Autodesk Fusion 360 part; units mm, degrees
(part 3 of 18)
  line L1811 (74.8364, -20.1454) -> (75.1219, -20.8347)
  line L1812 (79.0262, -16.9304) -> (78.3369, -16.6449)
  line L1813 (74.739, -19.4056) -> (74.8364, -20.1454)
  line L1814 (76.1681, -16.9304) -> (75.5761, -17.3846)
  line L1815 (80.3579, -18.6659) -> (80.0724, -17.9766)
  line L1816 (75.1219, -20.8347) -> (75.5761, -21.4267)
  line L1817 (78.3369, -16.6449) -> (77.5972, -16.5475)
  line L1818 (79.6182, -17.3846) -> (79.0262, -16.9304)
  line L1819 (75.1219, -17.9766) -> (74.8364, -18.6659)
  line L1820 (77.5972, -22.2638) -> (78.3369, -22.1664)
  line L1821 (75.5761, -21.4267) -> (76.1681, -21.8809)
  line L1822 (76.8574, -16.6449) -> (76.1681, -16.9304)
  line L1823 (80.3579, -20.1454) -> (80.4553, -19.4056)
  line L1824 (76.8574, -22.1664) -> (77.5972, -22.2638)
  line L1825 (76.1681, -21.8809) -> (76.8574, -22.1664)
  line L1826 (76.1681, -79.0564) -> (76.8574, -79.3419)
  line L1827 (80.3579, -75.8414) -> (80.0724, -75.1521)
  line L1828 (79.6182, -78.6022) -> (80.0724, -78.0102)
  line L1829 (79.0262, -79.0564) -> (79.6182, -78.6022)
  line L1830 (78.3369, -73.8204) -> (77.5972, -73.723)
  line L1831 (79.6182, -74.5601) -> (79.0262, -74.1059)
  line L1832 (74.739, -76.5812) -> (74.8364, -77.3209)
  line L1833 (76.1681, -74.1059) -> (75.5761, -74.5601)
  line L1834 (75.1219, -78.0102) -> (75.5761, -78.6022)
  line L1835 (74.8364, -77.3209) -> (75.1219, -78.0102)
  line L1836 (80.0724, -75.1521) -> (79.6182, -74.5601)
  line L1837 (80.4553, -76.5812) -> (80.3579, -75.8414)
  line L1838 (75.5761, -78.6022) -> (76.1681, -79.0564)
  line L1839 (80.3579, -77.3209) -> (80.4553, -76.5812)
  line L1840 (80.0724, -78.0102) -> (80.3579, -77.3209)
  line L1841 (75.1219, -75.1521) -> (74.8364, -75.8414)
  line L1842 (79.0262, -74.1059) -> (78.3369, -73.8204)
  line L1843 (77.5972, -79.4393) -> (78.3369, -79.3419)
  line L1844 (76.8574, -73.8204) -> (76.1681, -74.1059)
  line L1845 (74.8364, -75.8414) -> (74.739, -76.5812)
  line L1846 (75.5761, -74.5601) -> (75.1219, -75.1521)
  line L1847 (77.5972, -73.723) -> (76.8574, -73.8204)
  line L1848 (76.8574, -79.3419) -> (77.5972, -79.4393)
  line L1849 (78.3369, -79.3419) -> (79.0262, -79.0564)
  line L1850 (80.0724, -39.8847) -> (80.3579, -39.1954)
  line L1851 (76.1681, -35.9805) -> (75.5761, -36.4347)
  line L1852 (74.8364, -37.7159) -> (74.739, -38.4557)
  line L1853 (76.8574, -35.6949) -> (76.1681, -35.9805)
  line L1854 (80.4553, -38.4557) -> (80.3579, -37.7159)
  line L1855 (75.5761, -36.4347) -> (75.1219, -37.0266)
  line L1856 (75.1219, -37.0266) -> (74.8364, -37.7159)
  line L1857 (75.1219, -39.8847) -> (75.5761, -40.4767)
  line L1858 (79.0262, -40.9309) -> (79.6182, -40.4767)
  line L1859 (80.3579, -39.1954) -> (80.4553, -38.4557)
  line L1860 (80.3579, -37.7159) -> (80.0724, -37.0266)
  line L1861 (76.8574, -41.2164) -> (77.5972, -41.3138)
  line L1862 (77.5972, -35.5975) -> (76.8574, -35.6949)
  line L1863 (79.0262, -35.9805) -> (78.3369, -35.6949)
  line L1864 (77.5972, -41.3138) -> (78.3369, -41.2164)
  line L1865 (75.5761, -40.4767) -> (76.1681, -40.9309)
  line L1866 (78.3369, -41.2164) -> (79.0262, -40.9309)
  line L1867 (79.6182, -40.4767) -> (80.0724, -39.8847)
  line L1868 (78.3369, -35.6949) -> (77.5972, -35.5975)
  line L1869 (80.0724, -37.0266) -> (79.6182, -36.4347)
  line L1870 (79.6182, -36.4347) -> (79.0262, -35.9805)
  line L1871 (74.739, -38.4557) -> (74.8364, -39.1954)
  line L1872 (74.8364, -39.1954) -> (75.1219, -39.8847)
  line L1873 (76.1681, -40.9309) -> (76.8574, -41.2164)
  line L1874 (74.8364, -58.2582) -> (75.1219, -58.9475)
  line L1875 (79.0262, -59.9936) -> (79.6182, -59.5394)
  line L1876 (74.8364, -56.7787) -> (74.739, -57.5184)
  line L1877 (80.3579, -58.2582) -> (80.4553, -57.5184)
  line L1878 (79.6182, -59.5394) -> (80.0724, -58.9475)
  line L1879 (76.1681, -55.0432) -> (75.5761, -55.4974)
  line L1880 (75.1219, -58.9475) -> (75.5761, -59.5394)
  line L1881 (80.0724, -58.9475) -> (80.3579, -58.2582)
  line L1882 (74.739, -57.5184) -> (74.8364, -58.2582)
  line L1883 (75.1219, -56.0893) -> (74.8364, -56.7787)
  line L1884 (76.8574, -54.7577) -> (76.1681, -55.0432)
  line L1885 (78.3369, -54.7577) -> (77.5972, -54.6603)
  line L1886 (79.0262, -55.0432) -> (78.3369, -54.7577)
  line L1887 (75.5761, -55.4974) -> (75.1219, -56.0893)
  line L1888 (75.5761, -59.5394) -> (76.1681, -59.9936)
  line L1889 (77.5972, -54.6603) -> (76.8574, -54.7577)
  line L1890 (78.3369, -60.2792) -> (79.0262, -59.9936)
  line L1891 (77.5972, -60.3766) -> (78.3369, -60.2792)
  line L1892 (80.4553, -57.5184) -> (80.3579, -56.7787)
  line L1893 (80.3579, -56.7787) -> (80.0724, -56.0893)
  line L1894 (80.0724, -56.0893) -> (79.6182, -55.4974)
  line L1895 (79.6182, -55.4974) -> (79.0262, -55.0432)
  line L1896 (76.1681, -59.9936) -> (76.8574, -60.2792)
  line L1897 (76.8574, -60.2792) -> (77.5972, -60.3766)
  line L1898 (76.4348, -83.0626) -> (76.7075, -83.4708)
  line L1899 (76.4348, -82.0997) -> (76.339, -82.5812)
  line L1900 (76.7075, -81.6915) -> (76.4348, -82.0997)
  line L1901 (76.7075, -83.4708) -> (77.1157, -83.7435)
  line L1902 (78.0786, -81.4188) -> (77.5972, -81.323)
  line L1903 (77.1157, -83.7435) -> (77.5972, -83.8393)
  line L1904 (78.0786, -83.7435) -> (78.4868, -83.4708)
  line L1905 (78.4868, -83.4708) -> (78.7595, -83.0626)
  line L1906 (76.339, -82.5812) -> (76.4348, -83.0626)
  line L1907 (78.4868, -81.6915) -> (78.0786, -81.4188)
  line L1908 (78.7595, -82.0997) -> (78.4868, -81.6915)
  line L1909 (78.7595, -83.0626) -> (78.8553, -82.5812)
  line L1910 (77.1157, -81.4188) -> (76.7075, -81.6915)
  line L1911 (77.5972, -81.323) -> (77.1157, -81.4188)
  line L1912 (77.5972, -83.8393) -> (78.0786, -83.7435)
  line L1913 (78.8553, -82.5812) -> (78.7595, -82.0997)
  line L1914 (77.5972, -62.2603) -> (77.1157, -62.3561)
  line L1915 (76.4348, -63.037) -> (76.339, -63.5184)
  line L1916 (77.1157, -62.3561) -> (76.7075, -62.6288)
  line L1917 (78.0786, -62.3561) -> (77.5972, -62.2603)
  line L1918 (78.0786, -64.6808) -> (78.4868, -64.4081)
  line L1919 (78.8553, -63.5184) -> (78.7595, -63.037)
  line L1920 (76.339, -63.5184) -> (76.4348, -63.9999)
  line L1921 (76.7075, -62.6288) -> (76.4348, -63.037)
  line L1922 (78.7595, -63.037) -> (78.4868, -62.6288)
  line L1923 (77.1157, -64.6808) -> (77.5972, -64.7766)
  line L1924 (78.4868, -64.4081) -> (78.7595, -63.9999)
  line L1925 (78.4868, -62.6288) -> (78.0786, -62.3561)
  line L1926 (76.7075, -64.4081) -> (77.1157, -64.6808)
  line L1927 (78.7595, -63.9999) -> (78.8553, -63.5184)
  line L1928 (77.5972, -64.7766) -> (78.0786, -64.6808)
  line L1929 (76.4348, -63.9999) -> (76.7075, -64.4081)
  line L1930 (77.5972, -24.1475) -> (77.1157, -24.2433)
  line L1931 (76.7075, -24.516) -> (76.4348, -24.9242)
  line L1932 (78.7595, -24.9242) -> (78.4868, -24.516)
  line L1933 (78.7595, -25.8871) -> (78.8553, -25.4057)
  line L1934 (78.8553, -25.4057) -> (78.7595, -24.9242)
  line L1935 (77.1157, -24.2433) -> (76.7075, -24.516)
  line L1936 (77.5972, -26.6638) -> (78.0786, -26.568)
  line L1937 (76.4348, -25.8871) -> (76.7075, -26.2953)
  line L1938 (78.4868, -24.516) -> (78.0786, -24.2433)
  line L1939 (78.4868, -26.2953) -> (78.7595, -25.8871)
  line L1940 (76.339, -25.4057) -> (76.4348, -25.8871)
  line L1941 (78.0786, -24.2433) -> (77.5972, -24.1475)
  line L1942 (77.1157, -26.568) -> (77.5972, -26.6638)
  line L1943 (76.4348, -24.9242) -> (76.339, -25.4057)
  line L1944 (78.0786, -26.568) -> (78.4868, -26.2953)
  line L1945 (76.7075, -26.2953) -> (77.1157, -26.568)
  line L1946 (78.0786, -43.2933) -> (77.5972, -43.1975)
  line L1947 (77.1157, -43.2933) -> (76.7075, -43.566)
  line L1948 (76.7075, -45.3453) -> (77.1157, -45.6181)
  line L1949 (76.4348, -43.9742) -> (76.339, -44.4557)
  line L1950 (78.8553, -44.4557) -> (78.7595, -43.9742)
  line L1951 (76.339, -44.4557) -> (76.4348, -44.9372)
  line L1952 (76.4348, -44.9372) -> (76.7075, -45.3453)
  line L1953 (78.4868, -45.3453) -> (78.7595, -44.9372)
  line L1954 (77.5972, -45.7138) -> (78.0786, -45.6181)
  line L1955 (78.0786, -45.6181) -> (78.4868, -45.3453)
  line L1956 (78.7595, -44.9372) -> (78.8553, -44.4557)
  line L1957 (78.7595, -43.9742) -> (78.4868, -43.566)
  line L1958 (76.7075, -43.566) -> (76.4348, -43.9742)
  line L1959 (78.4868, -43.566) -> (78.0786, -43.2933)
  line L1960 (77.5972, -43.1975) -> (77.1157, -43.2933)
  line L1961 (77.1157, -45.6181) -> (77.5972, -45.7138)
  line L1962 (99.408, -20.1454) -> (99.5053, -19.4056)
  line L1963 (97.3869, -16.6449) -> (96.6472, -16.5475)
  line L1964 (99.5053, -19.4056) -> (99.408, -18.6659)
  line L1965 (93.789, -19.4056) -> (93.8864, -20.1454)
  line L1966 (96.6472, -22.2638) -> (97.3869, -22.1664)
  line L1967 (94.172, -17.9766) -> (93.8864, -18.6659)
  line L1968 (93.8864, -20.1454) -> (94.172, -20.8347)
  line L1969 (95.2181, -21.8809) -> (95.9075, -22.1664)
  line L1970 (99.408, -18.6659) -> (99.1224, -17.9766)
  line L1971 (93.8864, -18.6659) -> (93.789, -19.4056)
  line L1972 (99.1224, -17.9766) -> (98.6682, -17.3846)
  line L1973 (96.6472, -16.5475) -> (95.9075, -16.6449)
  line L1974 (94.172, -20.8347) -> (94.6262, -21.4267)
  line L1975 (97.3869, -22.1664) -> (98.0763, -21.8809)
  line L1976 (98.0763, -16.9304) -> (97.3869, -16.6449)
  line L1977 (95.9075, -16.6449) -> (95.2181, -16.9304)
  line L1978 (98.6682, -17.3846) -> (98.0763, -16.9304)
  line L1979 (99.1224, -20.8347) -> (99.408, -20.1454)
  line L1980 (94.6262, -21.4267) -> (95.2181, -21.8809)
  line L1981 (94.6262, -17.3846) -> (94.172, -17.9766)
  line L1982 (95.2181, -16.9304) -> (94.6262, -17.3846)
  line L1983 (95.9075, -22.1664) -> (96.6472, -22.2638)
  line L1984 (98.6682, -21.4267) -> (99.1224, -20.8347)
  line L1985 (98.0763, -21.8809) -> (98.6682, -21.4267)
  line L1986 (95.9075, -73.8204) -> (95.2181, -74.1059)
  line L1987 (96.6472, -73.723) -> (95.9075, -73.8204)
  line L1988 (95.2181, -74.1059) -> (94.6262, -74.5601)
  line L1989 (95.2181, -79.0564) -> (95.9075, -79.3419)
  line L1990 (96.6472, -79.4393) -> (97.3869, -79.3419)
  line L1991 (99.1224, -78.0102) -> (99.408, -77.3209)
  line L1992 (97.3869, -79.3419) -> (98.0763, -79.0564)
  line L1993 (94.6262, -78.6022) -> (95.2181, -79.0564)
  line L1994 (93.789, -76.5812) -> (93.8864, -77.3209)
  line L1995 (99.408, -77.3209) -> (99.5053, -76.5812)
  line L1996 (94.6262, -74.5601) -> (94.172, -75.1521)
  line L1997 (93.8864, -77.3209) -> (94.172, -78.0102)
  line L1998 (98.0763, -79.0564) -> (98.6682, -78.6022)
  line L1999 (93.8864, -75.8414) -> (93.789, -76.5812)
  line L2000 (98.6682, -78.6022) -> (99.1224, -78.0102)
  line L2001 (95.9075, -79.3419) -> (96.6472, -79.4393)
  line L2002 (98.0763, -74.1059) -> (97.3869, -73.8204)
  line L2003 (99.1224, -75.1521) -> (98.6682, -74.5601)
  line L2004 (94.172, -75.1521) -> (93.8864, -75.8414)
  line L2005 (97.3869, -73.8204) -> (96.6472, -73.723)
  line L2006 (99.5053, -76.5812) -> (99.408, -75.8414)
  line L2007 (94.172, -78.0102) -> (94.6262, -78.6022)
  line L2008 (98.6682, -74.5601) -> (98.0763, -74.1059)
  line L2009 (99.408, -75.8414) -> (99.1224, -75.1521)
  line L2010 (93.8864, -39.1954) -> (94.172, -39.8847)
  line L2011 (97.3869, -35.6949) -> (96.6472, -35.5975)
  line L2012 (98.0763, -35.9805) -> (97.3869, -35.6949)
  line L2013 (98.6682, -36.4347) -> (98.0763, -35.9805)
  line L2014 (97.3869, -41.2164) -> (98.0763, -40.9309)
  line L2015 (99.5053, -38.4557) -> (99.408, -37.7159)
  line L2016 (93.8864, -37.7159) -> (93.789, -38.4557)
  line L2017 (93.789, -38.4557) -> (93.8864, -39.1954)
  line L2018 (94.172, -37.0266) -> (93.8864, -37.7159)
  line L2019 (95.9075, -35.6949) -> (95.2181, -35.9805)
  line L2020 (94.6262, -40.4767) -> (95.2181, -40.9309)
  line L2021 (96.6472, -35.5975) -> (95.9075, -35.6949)
  line L2022 (95.2181, -35.9805) -> (94.6262, -36.4347)
  line L2023 (94.172, -39.8847) -> (94.6262, -40.4767)
  line L2024 (99.408, -37.7159) -> (99.1224, -37.0266)
  line L2025 (96.6472, -41.3138) -> (97.3869, -41.2164)
  line L2026 (95.2181, -40.9309) -> (95.9075, -41.2164)
  line L2027 (95.9075, -41.2164) -> (96.6472, -41.3138)
  line L2028 (99.408, -39.1954) -> (99.5053, -38.4557)
  line L2029 (94.6262, -36.4347) -> (94.172, -37.0266)
  line L2030 (99.1224, -39.8847) -> (99.408, -39.1954)
  line L2031 (98.6682, -40.4767) -> (99.1224, -39.8847)
  line L2032 (99.1224, -37.0266) -> (98.6682, -36.4347)
  line L2033 (98.0763, -40.9309) -> (98.6682, -40.4767)
  line L2034 (95.2181, -59.9936) -> (95.9075, -60.2792)
  line L2035 (99.408, -56.7787) -> (99.1224, -56.0893)
  line L2036 (93.8864, -58.2582) -> (94.172, -58.9475)
  line L2037 (98.0763, -59.9936) -> (98.6682, -59.5394)
  line L2038 (95.2181, -55.0432) -> (94.6262, -55.4974)
  line L2039 (97.3869, -60.2792) -> (98.0763, -59.9936)
  line L2040 (97.3869, -54.7577) -> (96.6472, -54.6603)
  line L2041 (94.6262, -55.4974) -> (94.172, -56.0893)
  line L2042 (93.789, -57.5184) -> (93.8864, -58.2582)
  line L2043 (99.1224, -56.0893) -> (98.6682, -55.4974)
  line L2044 (95.9075, -60.2792) -> (96.6472, -60.3766)
  line L2045 (99.1224, -58.9475) -> (99.408, -58.2582)
  line L2046 (98.6682, -55.4974) -> (98.0763, -55.0432)
  line L2047 (94.6262, -59.5394) -> (95.2181, -59.9936)
  line L2048 (96.6472, -60.3766) -> (97.3869, -60.2792)
  line L2049 (94.172, -56.0893) -> (93.8864, -56.7787)
  line L2050 (98.0763, -55.0432) -> (97.3869, -54.7577)
  line L2051 (99.5053, -57.5184) -> (99.408, -56.7787)
  line L2052 (99.408, -58.2582) -> (99.5053, -57.5184)
  line L2053 (96.6472, -54.6603) -> (95.9075, -54.7577)
  line L2054 (93.8864, -56.7787) -> (93.789, -57.5184)
  line L2055 (98.6682, -59.5394) -> (99.1224, -58.9475)
  line L2056 (94.172, -58.9475) -> (94.6262, -59.5394)
  line L2057 (95.9075, -54.7577) -> (95.2181, -55.0432)
  line L2058 (95.7576, -81.6915) -> (95.4848, -82.0997)
  line L2059 (97.9053, -82.5812) -> (97.8096, -82.0997)
  line L2060 (95.7576, -83.4708) -> (96.1657, -83.7435)
  line L2061 (97.5368, -83.4708) -> (97.8096, -83.0626)
  line L2062 (96.1657, -83.7435) -> (96.6472, -83.8393)
  line L2063 (97.8096, -83.0626) -> (97.9053, -82.5812)
  line L2064 (95.4848, -83.0626) -> (95.7576, -83.4708)
  line L2065 (97.1287, -81.4188) -> (96.6472, -81.323)
  line L2066 (97.8096, -82.0997) -> (97.5368, -81.6915)
  line L2067 (96.6472, -83.8393) -> (97.1287, -83.7435)
  line L2068 (96.1657, -81.4188) -> (95.7576, -81.6915)
  line L2069 (95.4848, -82.0997) -> (95.3891, -82.5812)
  line L2070 (95.3891, -82.5812) -> (95.4848, -83.0626)
  line L2071 (96.6472, -81.323) -> (96.1657, -81.4188)
  line L2072 (97.5368, -81.6915) -> (97.1287, -81.4188)
  line L2073 (97.1287, -83.7435) -> (97.5368, -83.4708)
  line L2074 (96.6472, -64.7766) -> (97.1287, -64.6808)
  line L2075 (95.7576, -62.6288) -> (95.4848, -63.037)
  line L2076 (97.1287, -62.3561) -> (96.6472, -62.2603)
  line L2077 (97.5368, -62.6288) -> (97.1287, -62.3561)
  line L2078 (95.3891, -63.5184) -> (95.4848, -63.9999)
  line L2079 (96.6472, -62.2603) -> (96.1657, -62.3561)
  line L2080 (97.8096, -63.9999) -> (97.9053, -63.5184)
  line L2081 (95.4848, -63.037) -> (95.3891, -63.5184)
  line L2082 (95.7576, -64.4081) -> (96.1657, -64.6808)
  line L2083 (97.9053, -63.5184) -> (97.8096, -63.037)
  line L2084 (95.4848, -63.9999) -> (95.7576, -64.4081)
  line L2085 (97.1287, -64.6808) -> (97.5368, -64.4081)
  line L2086 (97.8096, -63.037) -> (97.5368, -62.6288)
  line L2087 (96.1657, -62.3561) -> (95.7576, -62.6288)
  line L2088 (96.1657, -64.6808) -> (96.6472, -64.7766)
  line L2089 (97.5368, -64.4081) -> (97.8096, -63.9999)
  line L2090 (97.8096, -24.9242) -> (97.5368, -24.516)
  line L2091 (95.4848, -24.9242) -> (95.3891, -25.4057)
  line L2092 (95.3891, -25.4057) -> (95.4848, -25.8871)
  line L2093 (95.4848, -25.8871) -> (95.7576, -26.2953)
  line L2094 (97.9053, -25.4057) -> (97.8096, -24.9242)
  line L2095 (96.6472, -24.1475) -> (96.1657, -24.2433)
  line L2096 (95.7576, -24.516) -> (95.4848, -24.9242)
  line L2097 (97.5368, -26.2953) -> (97.8096, -25.8871)
  line L2098 (97.8096, -25.8871) -> (97.9053, -25.4057)
  line L2099 (96.1657, -24.2433) -> (95.7576, -24.516)
  line L2100 (97.1287, -26.568) -> (97.5368, -26.2953)
  line L2101 (96.6472, -26.6638) -> (97.1287, -26.568)
  line L2102 (97.1287, -24.2433) -> (96.6472, -24.1475)
  line L2103 (96.1657, -26.568) -> (96.6472, -26.6638)
  line L2104 (97.5368, -24.516) -> (97.1287, -24.2433)
  line L2105 (95.7576, -26.2953) -> (96.1657, -26.568)
  line L2106 (96.1657, -43.2933) -> (95.7576, -43.566)
  line L2107 (95.4848, -44.9372) -> (95.7576, -45.3453)
  line L2108 (95.4848, -43.9742) -> (95.3891, -44.4557)
  line L2109 (95.7576, -43.566) -> (95.4848, -43.9742)
  line L2110 (96.1657, -45.6181) -> (96.6472, -45.7138)
  line L2111 (97.1287, -45.6181) -> (97.5368, -45.3453)
  line L2112 (97.8096, -43.9742) -> (97.5368, -43.566)
  line L2113 (97.5368, -45.3453) -> (97.8096, -44.9372)
  line L2114 (96.6472, -45.7138) -> (97.1287, -45.6181)
  line L2115 (97.5368, -43.566) -> (97.1287, -43.2933)
  line L2116 (97.9053, -44.4557) -> (97.8096, -43.9742)
  line L2117 (97.1287, -43.2933) -> (96.6472, -43.1975)
  line L2118 (96.6472, -43.1975) -> (96.1657, -43.2933)
  line L2119 (95.7576, -45.3453) -> (96.1657, -45.6181)
  line L2120 (95.3891, -44.4557) -> (95.4848, -44.9372)
  line L2121 (97.8096, -44.9372) -> (97.9053, -44.4557)
  line L2122 (114.2682, -21.8809) -> (114.9575, -22.1664)
  line L2123 (113.222, -20.8347) -> (113.6762, -21.4267)
  line L2124 (112.9365, -18.6659) -> (112.8391, -19.4056)
  line L2125 (116.437, -16.6449) -> (115.6972, -16.5475)
  line L2126 (115.6972, -22.2638) -> (116.437, -22.1664)
  line L2127 (114.2682, -16.9304) -> (113.6762, -17.3846)
  line L2128 (117.1263, -21.8809) -> (117.7182, -21.4267)
  line L2129 (117.7182, -21.4267) -> (118.1725, -20.8347)
  line L2130 (117.1263, -16.9304) -> (116.437, -16.6449)
  line L2131 (115.6972, -16.5475) -> (114.9575, -16.6449)
  line L2132 (112.8391, -19.4056) -> (112.9365, -20.1454)
  line L2133 (113.222, -17.9766) -> (112.9365, -18.6659)
  line L2134 (118.1725, -17.9766) -> (117.7182, -17.3846)
  line L2135 (116.437, -22.1664) -> (117.1263, -21.8809)
  line L2136 (118.5554, -19.4056) -> (118.458, -18.6659)
  line L2137 (112.9365, -20.1454) -> (113.222, -20.8347)
  line L2138 (118.1725, -20.8347) -> (118.458, -20.1454)
  line L2139 (114.9575, -22.1664) -> (115.6972, -22.2638)
  line L2140 (113.6762, -17.3846) -> (113.222, -17.9766)
  line L2141 (113.6762, -21.4267) -> (114.2682, -21.8809)
  line L2142 (118.458, -20.1454) -> (118.5554, -19.4056)
  line L2143 (117.7182, -17.3846) -> (117.1263, -16.9304)
  line L2144 (118.458, -18.6659) -> (118.1725, -17.9766)
  line L2145 (114.9575, -16.6449) -> (114.2682, -16.9304)
  line L2146 (117.1263, -79.0564) -> (117.7182, -78.6022)
  line L2147 (113.6762, -74.5601) -> (113.222, -75.1521)
  line L2148 (118.5554, -76.5812) -> (118.458, -75.8414)
  line L2149 (117.1263, -74.1059) -> (116.437, -73.8204)
  line L2150 (114.9575, -73.8204) -> (114.2682, -74.1059)
  line L2151 (114.2682, -74.1059) -> (113.6762, -74.5601)
  line L2152 (117.7182, -78.6022) -> (118.1725, -78.0102)
  line L2153 (115.6972, -79.4393) -> (116.437, -79.3419)
  line L2154 (117.7182, -74.5601) -> (117.1263, -74.1059)
  line L2155 (118.1725, -78.0102) -> (118.458, -77.3209)
  line L2156 (112.9365, -75.8414) -> (112.8391, -76.5812)
  line L2157 (118.458, -77.3209) -> (118.5554, -76.5812)
  line L2158 (116.437, -73.8204) -> (115.6972, -73.723)
  line L2159 (113.222, -75.1521) -> (112.9365, -75.8414)
  line L2160 (118.458, -75.8414) -> (118.1725, -75.1521)
  line L2161 (113.222, -78.0102) -> (113.6762, -78.6022)
  line L2162 (113.6762, -78.6022) -> (114.2682, -79.0564)
  line L2163 (116.437, -79.3419) -> (117.1263, -79.0564)
  line L2164 (114.2682, -79.0564) -> (114.9575, -79.3419)
  line L2165 (118.1725, -75.1521) -> (117.7182, -74.5601)
  line L2166 (112.8391, -76.5812) -> (112.9365, -77.3209)
  line L2167 (115.6972, -73.723) -> (114.9575, -73.8204)
  line L2168 (114.9575, -79.3419) -> (115.6972, -79.4393)
  line L2169 (112.9365, -77.3209) -> (113.222, -78.0102)
  line L2170 (113.222, -37.0266) -> (112.9365, -37.7159)
  line L2171 (115.6972, -41.3138) -> (116.437, -41.2164)
  line L2172 (117.1263, -35.9805) -> (116.437, -35.6949)
  line L2173 (112.9365, -37.7159) -> (112.8391, -38.4557)
  line L2174 (114.9575, -41.2164) -> (115.6972, -41.3138)
  line L2175 (113.6762, -40.4767) -> (114.2682, -40.9309)
  line L2176 (117.7182, -36.4347) -> (117.1263, -35.9805)
  line L2177 (118.458, -39.1954) -> (118.5554, -38.4557)
  line L2178 (118.458, -37.7159) -> (118.1725, -37.0266)
  line L2179 (118.1725, -39.8847) -> (118.458, -39.1954)
  line L2180 (114.2682, -35.9805) -> (113.6762, -36.4347)
  line L2181 (113.222, -39.8847) -> (113.6762, -40.4767)
  line L2182 (118.5554, -38.4557) -> (118.458, -37.7159)
  line L2183 (116.437, -41.2164) -> (117.1263, -40.9309)
  line L2184 (118.1725, -37.0266) -> (117.7182, -36.4347)
  line L2185 (117.1263, -40.9309) -> (117.7182, -40.4767)
  line L2186 (117.7182, -40.4767) -> (118.1725, -39.8847)
  line L2187 (116.437, -35.6949) -> (115.6972, -35.5975)
  line L2188 (114.9575, -35.6949) -> (114.2682, -35.9805)
  line L2189 (112.9365, -39.1954) -> (113.222, -39.8847)
  line L2190 (113.6762, -36.4347) -> (113.222, -37.0266)
  line L2191 (115.6972, -35.5975) -> (114.9575, -35.6949)
  line L2192 (112.8391, -38.4557) -> (112.9365, -39.1954)
  line L2193 (114.2682, -40.9309) -> (114.9575, -41.2164)
  line L2194 (117.7182, -59.5394) -> (118.1725, -58.9475)
  line L2195 (114.2682, -55.0432) -> (113.6762, -55.4974)
  line L2196 (117.7182, -55.4974) -> (117.1263, -55.0432)
  line L2197 (118.458, -56.7787) -> (118.1725, -56.0893)
  line L2198 (112.9365, -56.7787) -> (112.8391, -57.5184)
  line L2199 (117.1263, -55.0432) -> (116.437, -54.7577)
  line L2200 (115.6972, -54.6603) -> (114.9575, -54.7577)
  line L2201 (114.9575, -54.7577) -> (114.2682, -55.0432)
  line L2202 (113.6762, -55.4974) -> (113.222, -56.0893)
  line L2203 (117.1263, -59.9936) -> (117.7182, -59.5394)
  line L2204 (116.437, -60.2792) -> (117.1263, -59.9936)
  line L2205 (114.2682, -59.9936) -> (114.9575, -60.2792)
  line L2206 (114.9575, -60.2792) -> (115.6972, -60.3766)
  line L2207 (118.1725, -56.0893) -> (117.7182, -55.4974)
  line L2208 (113.6762, -59.5394) -> (114.2682, -59.9936)
  line L2209 (112.8391, -57.5184) -> (112.9365, -58.2582)
  line L2210 (113.222, -58.9475) -> (113.6762, -59.5394)
  line L2211 (112.9365, -58.2582) -> (113.222, -58.9475)
  line L2212 (118.5554, -57.5184) -> (118.458, -56.7787)
  line L2213 (118.458, -58.2582) -> (118.5554, -57.5184)
  line L2214 (118.1725, -58.9475) -> (118.458, -58.2582)
  line L2215 (115.6972, -60.3766) -> (116.437, -60.2792)
  line L2216 (113.222, -56.0893) -> (112.9365, -56.7787)
  line L2217 (116.437, -54.7577) -> (115.6972, -54.6603)
  line L2218 (115.6972, -81.323) -> (115.2158, -81.4188)
  line L2219 (115.2158, -83.7435) -> (115.6972, -83.8393)
  line L2220 (116.5869, -81.6915) -> (116.1787, -81.4188)
  line L2221 (116.8596, -82.0997) -> (116.5869, -81.6915)
  line L2222 (114.8076, -81.6915) -> (114.5349, -82.0997)
  line L2223 (115.2158, -81.4188) -> (114.8076, -81.6915)
  line L2224 (114.5349, -82.0997) -> (114.4391, -82.5812)
  line L2225 (116.1787, -81.4188) -> (115.6972, -81.323)
  line L2226 (116.1787, -83.7435) -> (116.5869, -83.4708)
  line L2227 (115.6972, -83.8393) -> (116.1787, -83.7435)
  line L2228 (114.4391, -82.5812) -> (114.5349, -83.0626)
  line L2229 (116.5869, -83.4708) -> (116.8596, -83.0626)
  line L2230 (116.8596, -83.0626) -> (116.9554, -82.5812)
  line L2231 (114.8076, -83.4708) -> (115.2158, -83.7435)
  line L2232 (116.9554, -82.5812) -> (116.8596, -82.0997)
  line L2233 (114.5349, -83.0626) -> (114.8076, -83.4708)
  line L2234 (116.5869, -64.4081) -> (116.8596, -63.9999)
  line L2235 (115.2158, -62.3561) -> (114.8076, -62.6288)
  line L2236 (114.5349, -63.9999) -> (114.8076, -64.4081)
  line L2237 (116.9554, -63.5184) -> (116.8596, -63.037)
  line L2238 (115.2158, -64.6808) -> (115.6972, -64.7766)
  line L2239 (114.8076, -62.6288) -> (114.5349, -63.037)
  line L2240 (116.8596, -63.9999) -> (116.9554, -63.5184)
  line L2241 (116.8596, -63.037) -> (116.5869, -62.6288)
  line L2242 (114.8076, -64.4081) -> (115.2158, -64.6808)
  line L2243 (115.6972, -62.2603) -> (115.2158, -62.3561)
  line L2244 (114.4391, -63.5184) -> (114.5349, -63.9999)
  line L2245 (116.5869, -62.6288) -> (116.1787, -62.3561)
  line L2246 (116.1787, -64.6808) -> (116.5869, -64.4081)
  line L2247 (114.5349, -63.037) -> (114.4391, -63.5184)
  line L2248 (116.1787, -62.3561) -> (115.6972, -62.2603)
  line L2249 (115.6972, -64.7766) -> (116.1787, -64.6808)
  line L2250 (116.9554, -25.4057) -> (116.8596, -24.9242)
  line L2251 (114.4391, -25.4057) -> (114.5349, -25.8871)
  line L2252 (114.8076, -26.2953) -> (115.2158, -26.568)
  line L2253 (116.5869, -24.516) -> (116.1787, -24.2433)
  line L2254 (114.5349, -24.9242) -> (114.4391, -25.4057)
  line L2255 (115.2158, -24.2433) -> (114.8076, -24.516)
  line L2256 (116.8596, -24.9242) -> (116.5869, -24.516)
  line L2257 (116.8596, -25.8871) -> (116.9554, -25.4057)
  line L2258 (116.1787, -24.2433) -> (115.6972, -24.1475)
  line L2259 (115.6972, -24.1475) -> (115.2158, -24.2433)
  line L2260 (116.5869, -26.2953) -> (116.8596, -25.8871)
  line L2261 (114.8076, -24.516) -> (114.5349, -24.9242)
  line L2262 (116.1787, -26.568) -> (116.5869, -26.2953)
  line L2263 (115.6972, -26.6638) -> (116.1787, -26.568)
  line L2264 (114.5349, -25.8871) -> (114.8076, -26.2953)
  line L2265 (115.2158, -26.568) -> (115.6972, -26.6638)
  line L2266 (115.6972, -45.7138) -> (116.1787, -45.6181)
  line L2267 (116.1787, -43.2933) -> (115.6972, -43.1975)
  line L2268 (116.5869, -45.3453) -> (116.8596, -44.9372)
  line L2269 (114.8076, -43.566) -> (114.5349, -43.9742)
  line L2270 (115.6972, -43.1975) -> (115.2158, -43.2933)
  line L2271 (114.8076, -45.3453) -> (115.2158, -45.6181)
  line L2272 (114.4391, -44.4557) -> (114.5349, -44.9372)
  line L2273 (114.5349, -43.9742) -> (114.4391, -44.4557)
  line L2274 (116.8596, -43.9742) -> (116.5869, -43.566)
  line L2275 (114.5349, -44.9372) -> (114.8076, -45.3453)
  line L2276 (115.2158, -45.6181) -> (115.6972, -45.7138)
  line L2277 (116.8596, -44.9372) -> (116.9554, -44.4557)
  line L2278 (116.1787, -45.6181) -> (116.5869, -45.3453)
  line L2279 (115.2158, -43.2933) -> (114.8076, -43.566)
  line L2280 (116.9554, -44.4557) -> (116.8596, -43.9742)
  line L2281 (116.5869, -43.566) -> (116.1787, -43.2933)
  line L2282 (137.2225, -20.8347) -> (137.508, -20.1454)
  line L2283 (132.272, -17.9766) -> (131.9865, -18.6659)
  line L2284 (136.1763, -16.9304) -> (135.487, -16.6449)
  line L2285 (132.272, -20.8347) -> (132.7263, -21.4267)
  line L2286 (135.487, -22.1664) -> (136.1763, -21.8809)
  line L2287 (137.508, -20.1454) -> (137.6054, -19.4056)
  line L2288 (134.7473, -16.5475) -> (134.0075, -16.6449)
  line L2289 (134.7473, -22.2638) -> (135.487, -22.1664)
  line L2290 (131.9865, -18.6659) -> (131.8891, -19.4056)
  line L2291 (133.3182, -21.8809) -> (134.0075, -22.1664)
  line L2292 (137.2225, -17.9766) -> (136.7683, -17.3846)
  line L2293 (136.1763, -21.8809) -> (136.7683, -21.4267)
  line L2294 (136.7683, -21.4267) -> (137.2225, -20.8347)
  line L2295 (132.7263, -21.4267) -> (133.3182, -21.8809)
  line L2296 (131.9865, -20.1454) -> (132.272, -20.8347)
  line L2297 (131.8891, -19.4056) -> (131.9865, -20.1454)
  line L2298 (136.7683, -17.3846) -> (136.1763, -16.9304)
  line L2299 (134.0075, -16.6449) -> (133.3182, -16.9304)
  line L2300 (132.7263, -17.3846) -> (132.272, -17.9766)
  line L2301 (137.508, -18.6659) -> (137.2225, -17.9766)
  line L2302 (135.487, -16.6449) -> (134.7473, -16.5475)
  line L2303 (134.0075, -22.1664) -> (134.7473, -22.2638)
  line L2304 (137.6054, -19.4056) -> (137.508, -18.6659)
  line L2305 (133.3182, -16.9304) -> (132.7263, -17.3846)
  line L2306 (134.7473, -73.723) -> (134.0075, -73.8204)
  line L2307 (132.7263, -78.6022) -> (133.3182, -79.0564)
  line L2308 (134.0075, -73.8204) -> (133.3182, -74.1059)
  line L2309 (135.487, -73.8204) -> (134.7473, -73.723)
  line L2310 (131.8891, -76.5812) -> (131.9865, -77.3209)
  line L2311 (134.0075, -79.3419) -> (134.7473, -79.4393)
  line L2312 (131.9865, -77.3209) -> (132.272, -78.0102)
  line L2313 (135.487, -79.3419) -> (136.1763, -79.0564)
  line L2314 (136.7683, -78.6022) -> (137.2225, -78.0102)
  line L2315 (132.272, -78.0102) -> (132.7263, -78.6022)
  line L2316 (133.3182, -79.0564) -> (134.0075, -79.3419)
  line L2317 (136.1763, -74.1059) -> (135.487, -73.8204)
  line L2318 (131.9865, -75.8414) -> (131.8891, -76.5812)
  line L2319 (137.508, -75.8414) -> (137.2225, -75.1521)
  line L2320 (132.7263, -74.5601) -> (132.272, -75.1521)
  line L2321 (137.2225, -78.0102) -> (137.508, -77.3209)
  line L2322 (137.2225, -75.1521) -> (136.7683, -74.5601)
  line L2323 (136.7683, -74.5601) -> (136.1763, -74.1059)
  line L2324 (136.1763, -79.0564) -> (136.7683, -78.6022)
  line L2325 (133.3182, -74.1059) -> (132.7263, -74.5601)
  line L2326 (132.272, -75.1521) -> (131.9865, -75.8414)
  line L2327 (137.6054, -76.5812) -> (137.508, -75.8414)
  line L2328 (134.7473, -79.4393) -> (135.487, -79.3419)
  line L2329 (137.508, -77.3209) -> (137.6054, -76.5812)
  line L2330 (137.2225, -37.0266) -> (136.7683, -36.4347)
  line L2331 (137.508, -39.1954) -> (137.6054, -38.4557)
  line L2332 (136.7683, -36.4347) -> (136.1763, -35.9805)
  line L2333 (134.7473, -41.3138) -> (135.487, -41.2164)
  line L2334 (137.2225, -39.8847) -> (137.508, -39.1954)
  line L2335 (131.9865, -37.7159) -> (131.8891, -38.4557)
  line L2336 (132.7263, -36.4347) -> (132.272, -37.0266)
  line L2337 (134.0075, -41.2164) -> (134.7473, -41.3138)
  line L2338 (136.1763, -40.9309) -> (136.7683, -40.4767)
  line L2339 (131.9865, -39.1954) -> (132.272, -39.8847)
  line L2340 (137.6054, -38.4557) -> (137.508, -37.7159)
  line L2341 (135.487, -35.6949) -> (134.7473, -35.5975)
  line L2342 (132.7263, -40.4767) -> (133.3182, -40.9309)
  line L2343 (134.0075, -35.6949) -> (133.3182, -35.9805)
  line L2344 (135.487, -41.2164) -> (136.1763, -40.9309)
  line L2345 (133.3182, -40.9309) -> (134.0075, -41.2164)
  line L2346 (136.7683, -40.4767) -> (137.2225, -39.8847)
  line L2347 (132.272, -37.0266) -> (131.9865, -37.7159)
  line L2348 (133.3182, -35.9805) -> (132.7263, -36.4347)
  line L2349 (137.508, -37.7159) -> (137.2225, -37.0266)
  line L2350 (131.8891, -38.4557) -> (131.9865, -39.1954)
  line L2351 (134.7473, -35.5975) -> (134.0075, -35.6949)
  line L2352 (136.1763, -35.9805) -> (135.487, -35.6949)
  line L2353 (132.272, -39.8847) -> (132.7263, -40.4767)
  line L2354 (132.7263, -59.5394) -> (133.3182, -59.9936)
  line L2355 (137.2225, -58.9475) -> (137.508, -58.2582)
  line L2356 (136.7683, -59.5394) -> (137.2225, -58.9475)
  line L2357 (134.7473, -60.3766) -> (135.487, -60.2792)
  line L2358 (131.8891, -57.5184) -> (131.9865, -58.2582)
  line L2359 (133.3182, -59.9936) -> (134.0075, -60.2792)
  line L2360 (132.272, -56.0893) -> (131.9865, -56.7787)
  line L2361 (134.0075, -60.2792) -> (134.7473, -60.3766)
  line L2362 (131.9865, -56.7787) -> (131.8891, -57.5184)
  line L2363 (137.508, -56.7787) -> (137.2225, -56.0893)
  line L2364 (135.487, -60.2792) -> (136.1763, -59.9936)
  line L2365 (136.1763, -55.0432) -> (135.487, -54.7577)
  line L2366 (133.3182, -55.0432) -> (132.7263, -55.4974)
  line L2367 (137.6054, -57.5184) -> (137.508, -56.7787)
  line L2368 (136.1763, -59.9936) -> (136.7683, -59.5394)
  line L2369 (132.7263, -55.4974) -> (132.272, -56.0893)
  line L2370 (132.272, -58.9475) -> (132.7263, -59.5394)
  line L2371 (137.2225, -56.0893) -> (136.7683, -55.4974)
  line L2372 (134.7473, -54.6603) -> (134.0075, -54.7577)
  line L2373 (137.508, -58.2582) -> (137.6054, -57.5184)
  line L2374 (131.9865, -58.2582) -> (132.272, -58.9475)
  line L2375 (134.0075, -54.7577) -> (133.3182, -55.0432)
  line L2376 (136.7683, -55.4974) -> (136.1763, -55.0432)
  line L2377 (135.487, -54.7577) -> (134.7473, -54.6603)
  line L2378 (133.8576, -83.4708) -> (134.2658, -83.7435)
  line L2379 (134.2658, -83.7435) -> (134.7473, -83.8393)
  line L2380 (133.4891, -82.5812) -> (133.5849, -83.0626)
  line L2381 (133.5849, -83.0626) -> (133.8576, -83.4708)
  line L2382 (135.6369, -83.4708) -> (135.9096, -83.0626)
  line L2383 (136.0054, -82.5812) -> (135.9096, -82.0997)
  line L2384 (134.2658, -81.4188) -> (133.8576, -81.6915)
  line L2385 (133.8576, -81.6915) -> (133.5849, -82.0997)
  line L2386 (133.5849, -82.0997) -> (133.4891, -82.5812)
  line L2387 (135.9096, -82.0997) -> (135.6369, -81.6915)
  line L2388 (134.7473, -81.323) -> (134.2658, -81.4188)
  line L2389 (135.2287, -81.4188) -> (134.7473, -81.323)
  line L2390 (135.6369, -81.6915) -> (135.2287, -81.4188)
  line L2391 (135.2287, -83.7435) -> (135.6369, -83.4708)
  line L2392 (134.7473, -83.8393) -> (135.2287, -83.7435)
  line L2393 (135.9096, -83.0626) -> (136.0054, -82.5812)
  line L2394 (135.2287, -64.6808) -> (135.6369, -64.4081)
  line L2395 (135.6369, -64.4081) -> (135.9096, -63.9999)
  line L2396 (135.6369, -62.6288) -> (135.2287, -62.3561)
  line L2397 (133.8576, -62.6288) -> (133.5849, -63.037)
  line L2398 (134.2658, -62.3561) -> (133.8576, -62.6288)
  line L2399 (135.9096, -63.037) -> (135.6369, -62.6288)
  line L2400 (136.0054, -63.5184) -> (135.9096, -63.037)
  line L2401 (133.4891, -63.5184) -> (133.5849, -63.9999)
  line L2402 (134.7473, -62.2603) -> (134.2658, -62.3561)
  line L2403 (133.5849, -63.037) -> (133.4891, -63.5184)
  line L2404 (135.9096, -63.9999) -> (136.0054, -63.5184)
  line L2405 (133.8576, -64.4081) -> (134.2658, -64.6808)
  line L2406 (135.2287, -62.3561) -> (134.7473, -62.2603)
  line L2407 (134.2658, -64.6808) -> (134.7473, -64.7766)
  line L2408 (134.7473, -64.7766) -> (135.2287, -64.6808)
  line L2409 (133.5849, -63.9999) -> (133.8576, -64.4081)
  line L2410 (133.4891, -25.4057) -> (133.5849, -25.8871)
  line L2411 (135.6369, -26.2953) -> (135.9096, -25.8871)
  line L2412 (134.7473, -24.1475) -> (134.2658, -24.2433)
  line L2413 (136.0054, -25.4057) -> (135.9096, -24.9242)
  line L2414 (135.9096, -25.8871) -> (136.0054, -25.4057)
  line L2415 (134.2658, -26.568) -> (134.7473, -26.6638)
  line L2416 (134.7473, -26.6638) -> (135.2287, -26.568)
  line L2417 (133.5849, -25.8871) -> (133.8576, -26.2953)
  line L2418 (135.9096, -24.9242) -> (135.6369, -24.516)
  line L2419 (135.2287, -26.568) -> (135.6369, -26.2953)
  line L2420 (135.6369, -24.516) -> (135.2287, -24.2433)
  line L2421 (133.8576, -24.516) -> (133.5849, -24.9242)
  line L2422 (133.5849, -24.9242) -> (133.4891, -25.4057)
  line L2423 (134.2658, -24.2433) -> (133.8576, -24.516)
  line L2424 (135.2287, -24.2433) -> (134.7473, -24.1475)
  line L2425 (133.8576, -26.2953) -> (134.2658, -26.568)
  line L2426 (134.7473, -43.1975) -> (134.2658, -43.2933)
  line L2427 (133.5849, -44.9372) -> (133.8576, -45.3453)
  line L2428 (136.0054, -44.4557) -> (135.9096, -43.9742)
  line L2429 (133.4891, -44.4557) -> (133.5849, -44.9372)
  line L2430 (133.8576, -43.566) -> (133.5849, -43.9742)
  line L2431 (135.9096, -43.9742) -> (135.6369, -43.566)
  line L2432 (135.6369, -45.3453) -> (135.9096, -44.9372)
  line L2433 (133.8576, -45.3453) -> (134.2658, -45.6181)
  line L2434 (134.2658, -45.6181) -> (134.7473, -45.7138)
  line L2435 (134.2658, -43.2933) -> (133.8576, -43.566)
  line L2436 (133.5849, -43.9742) -> (133.4891, -44.4557)
  line L2437 (135.9096, -44.9372) -> (136.0054, -44.4557)
  line L2438 (134.7473, -45.7138) -> (135.2287, -45.6181)
  line L2439 (135.2287, -45.6181) -> (135.6369, -45.3453)
  line L2440 (135.6369, -43.566) -> (135.2287, -43.2933)
  line L2441 (135.2287, -43.2933) -> (134.7473, -43.1975)
  line L2442 (153.0576, -22.1664) -> (153.7973, -22.2638)
  line L2443 (154.5371, -22.1664) -> (155.2264, -21.8809)
  line L2444 (156.5581, -18.6659) -> (156.2725, -17.9766)
  line L2445 (153.7973, -16.5475) -> (153.0576, -16.6449)
  line L2446 (150.9392, -19.4056) -> (151.0366, -20.1454)
  line L2447 (152.3682, -16.9304) -> (151.7763, -17.3846)
  line L2448 (151.0366, -20.1454) -> (151.3221, -20.8347)
  line L2449 (156.6555, -19.4056) -> (156.5581, -18.6659)
  line L2450 (156.2725, -20.8347) -> (156.5581, -20.1454)
  line L2451 (151.7763, -17.3846) -> (151.3221, -17.9766)
  line L2452 (151.0366, -18.6659) -> (150.9392, -19.4056)
  line L2453 (153.0576, -16.6449) -> (152.3682, -16.9304)
  line L2454 (155.8183, -17.3846) -> (155.2264, -16.9304)
  line L2455 (152.3682, -21.8809) -> (153.0576, -22.1664)
  line L2456 (156.2725, -17.9766) -> (155.8183, -17.3846)
  line L2457 (155.8183, -21.4267) -> (156.2725, -20.8347)
  line L2458 (155.2264, -16.9304) -> (154.5371, -16.6449)
  line L2459 (151.3221, -20.8347) -> (151.7763, -21.4267)
  line L2460 (153.7973, -22.2638) -> (154.5371, -22.1664)
  line L2461 (155.2264, -21.8809) -> (155.8183, -21.4267)
  line L2462 (151.3221, -17.9766) -> (151.0366, -18.6659)
  line L2463 (154.5371, -16.6449) -> (153.7973, -16.5475)
  line L2464 (156.5581, -20.1454) -> (156.6555, -19.4056)
  line L2465 (151.7763, -21.4267) -> (152.3682, -21.8809)
  line L2466 (151.7763, -74.5601) -> (151.3221, -75.1521)
  line L2467 (155.2264, -74.1059) -> (154.5371, -73.8204)
  line L2468 (155.8183, -74.5601) -> (155.2264, -74.1059)
  line L2469 (156.5581, -77.3209) -> (156.6555, -76.5812)
  line L2470 (156.2725, -75.1521) -> (155.8183, -74.5601)
  line L2471 (151.0366, -77.3209) -> (151.3221, -78.0102)
  line L2472 (153.0576, -73.8204) -> (152.3682, -74.1059)
  line L2473 (155.2264, -79.0564) -> (155.8183, -78.6022)
  line L2474 (153.7973, -79.4393) -> (154.5371, -79.3419)
  line L2475 (156.5581, -75.8414) -> (156.2725, -75.1521)
  line L2476 (153.7973, -73.723) -> (153.0576, -73.8204)
  line L2477 (152.3682, -74.1059) -> (151.7763, -74.5601)
  line L2478 (150.9392, -76.5812) -> (151.0366, -77.3209)
  line L2479 (156.6555, -76.5812) -> (156.5581, -75.8414)
  line L2480 (153.0576, -79.3419) -> (153.7973, -79.4393)
  line L2481 (151.7763, -78.6022) -> (152.3682, -79.0564)
  line L2482 (154.5371, -73.8204) -> (153.7973, -73.723)
  line L2483 (151.0366, -75.8414) -> (150.9392, -76.5812)
  line L2484 (151.3221, -75.1521) -> (151.0366, -75.8414)
  line L2485 (154.5371, -79.3419) -> (155.2264, -79.0564)
  line L2486 (152.3682, -79.0564) -> (153.0576, -79.3419)
  line L2487 (156.2725, -78.0102) -> (156.5581, -77.3209)
  line L2488 (155.8183, -78.6022) -> (156.2725, -78.0102)
  line L2489 (151.3221, -78.0102) -> (151.7763, -78.6022)
  line L2490 (153.7973, -35.5975) -> (153.0576, -35.6949)
  line L2491 (156.2725, -37.0266) -> (155.8183, -36.4347)
  line L2492 (151.0366, -37.7159) -> (150.9392, -38.4557)
  line L2493 (155.2264, -40.9309) -> (155.8183, -40.4767)
  line L2494 (152.3682, -40.9309) -> (153.0576, -41.2164)
  line L2495 (154.5371, -41.2164) -> (155.2264, -40.9309)
  line L2496 (151.7763, -40.4767) -> (152.3682, -40.9309)
  line L2497 (151.3221, -37.0266) -> (151.0366, -37.7159)
  line L2498 (151.7763, -36.4347) -> (151.3221, -37.0266)
  line L2499 (151.3221, -39.8847) -> (151.7763, -40.4767)
  line L2500 (156.5581, -39.1954) -> (156.6555, -38.4557)
  line L2501 (153.7973, -41.3138) -> (154.5371, -41.2164)
  line L2502 (156.6555, -38.4557) -> (156.5581, -37.7159)
  line L2503 (156.5581, -37.7159) -> (156.2725, -37.0266)
  line L2504 (156.2725, -39.8847) -> (156.5581, -39.1954)
  line L2505 (150.9392, -38.4557) -> (151.0366, -39.1954)
  line L2506 (155.2264, -35.9805) -> (154.5371, -35.6949)
  line L2507 (151.0366, -39.1954) -> (151.3221, -39.8847)
  line L2508 (155.8183, -40.4767) -> (156.2725, -39.8847)
  line L2509 (155.8183, -36.4347) -> (155.2264, -35.9805)
  line L2510 (154.5371, -35.6949) -> (153.7973, -35.5975)
  line L2511 (153.0576, -41.2164) -> (153.7973, -41.3138)
  line L2512 (153.0576, -35.6949) -> (152.3682, -35.9805)
  line L2513 (152.3682, -35.9805) -> (151.7763, -36.4347)
  line L2514 (151.3221, -56.0893) -> (151.0366, -56.7787)
  line L2515 (156.5581, -56.7787) -> (156.2725, -56.0893)
  line L2516 (153.0576, -54.7577) -> (152.3682, -55.0432)
  line L2517 (150.9392, -57.5184) -> (151.0366, -58.2582)
  line L2518 (152.3682, -59.9936) -> (153.0576, -60.2792)
  line L2519 (153.7973, -54.6603) -> (153.0576, -54.7577)
  line L2520 (154.5371, -54.7577) -> (153.7973, -54.6603)
  line L2521 (151.3221, -58.9475) -> (151.7763, -59.5394)
  line L2522 (154.5371, -60.2792) -> (155.2264, -59.9936)
  line L2523 (151.0366, -56.7787) -> (150.9392, -57.5184)
  line L2524 (155.8183, -55.4974) -> (155.2264, -55.0432)
  line L2525 (156.5581, -58.2582) -> (156.6555, -57.5184)
  line L2526 (156.6555, -57.5184) -> (156.5581, -56.7787)
  line L2527 (153.7973, -60.3766) -> (154.5371, -60.2792)
  line L2528 (156.2725, -56.0893) -> (155.8183, -55.4974)
  line L2529 (153.0576, -60.2792) -> (153.7973, -60.3766)
  line L2530 (151.7763, -55.4974) -> (151.3221, -56.0893)
  line L2531 (151.0366, -58.2582) -> (151.3221, -58.9475)
  line L2532 (156.2725, -58.9475) -> (156.5581, -58.2582)
  line L2533 (155.8183, -59.5394) -> (156.2725, -58.9475)
  line L2534 (151.7763, -59.5394) -> (152.3682, -59.9936)
  line L2535 (155.2264, -59.9936) -> (155.8183, -59.5394)
  line L2536 (152.3682, -55.0432) -> (151.7763, -55.4974)
  line L2537 (155.2264, -55.0432) -> (154.5371, -54.7577)
  line L2538 (154.6869, -81.6915) -> (154.2788, -81.4188)
  line L2539 (152.5392, -82.5812) -> (152.6349, -83.0626)
  line L2540 (154.2788, -83.7435) -> (154.6869, -83.4708)
  line L2541 (153.3158, -83.7435) -> (153.7973, -83.8393)
  line L2542 (152.6349, -83.0626) -> (152.9077, -83.4708)
  line L2543 (152.9077, -81.6915) -> (152.6349, -82.0997)
  line L2544 (152.9077, -83.4708) -> (153.3158, -83.7435)
  line L2545 (154.2788, -81.4188) -> (153.7973, -81.323)
  line L2546 (154.6869, -83.4708) -> (154.9597, -83.0626)
  line L2547 (153.7973, -81.323) -> (153.3158, -81.4188)
  line L2548 (153.3158, -81.4188) -> (152.9077, -81.6915)
  line L2549 (153.7973, -83.8393) -> (154.2788, -83.7435)
  line L2550 (152.6349, -82.0997) -> (152.5392, -82.5812)
  line L2551 (154.9597, -82.0997) -> (154.6869, -81.6915)
  line L2552 (154.9597, -83.0626) -> (155.0554, -82.5812)
  line L2553 (155.0554, -82.5812) -> (154.9597, -82.0997)
  line L2554 (155.0554, -63.5184) -> (154.9597, -63.037)
  line L2555 (154.6869, -64.4081) -> (154.9597, -63.9999)
  line L2556 (154.2788, -64.6808) -> (154.6869, -64.4081)
  line L2557 (153.3158, -64.6808) -> (153.7973, -64.7766)
  line L2558 (153.7973, -62.2603) -> (153.3158, -62.3561)
  line L2559 (152.5392, -63.5184) -> (152.6349, -63.9999)
  line L2560 (153.3158, -62.3561) -> (152.9077, -62.6288)
  line L2561 (152.9077, -62.6288) -> (152.6349, -63.037)
  line L2562 (154.9597, -63.9999) -> (155.0554, -63.5184)
  line L2563 (152.6349, -63.9999) -> (152.9077, -64.4081)
  line L2564 (154.6869, -62.6288) -> (154.2788, -62.3561)
  line L2565 (154.9597, -63.037) -> (154.6869, -62.6288)
  line L2566 (153.7973, -64.7766) -> (154.2788, -64.6808)
  line L2567 (152.9077, -64.4081) -> (153.3158, -64.6808)
  line L2568 (154.2788, -62.3561) -> (153.7973, -62.2603)
  line L2569 (152.6349, -63.037) -> (152.5392, -63.5184)
  line L2570 (154.2788, -24.2433) -> (153.7973, -24.1475)
  line L2571 (154.2788, -26.568) -> (154.6869, -26.2953)
  line L2572 (152.6349, -24.9242) -> (152.5392, -25.4057)
  line L2573 (152.5392, -25.4057) -> (152.6349, -25.8871)
  line L2574 (154.6869, -24.516) -> (154.2788, -24.2433)
  line L2575 (153.7973, -24.1475) -> (153.3158, -24.2433)
  line L2576 (154.9597, -25.8871) -> (155.0554, -25.4057)
  line L2577 (152.9077, -24.516) -> (152.6349, -24.9242)
  line L2578 (154.6869, -26.2953) -> (154.9597, -25.8871)
  line L2579 (154.9597, -24.9242) -> (154.6869, -24.516)
  line L2580 (153.7973, -26.6638) -> (154.2788, -26.568)
  line L2581 (152.6349, -25.8871) -> (152.9077, -26.2953)
  line L2582 (152.9077, -26.2953) -> (153.3158, -26.568)
  line L2583 (155.0554, -25.4057) -> (154.9597, -24.9242)
  line L2584 (153.3158, -24.2433) -> (152.9077, -24.516)
  line L2585 (153.3158, -26.568) -> (153.7973, -26.6638)
  line L2586 (153.3158, -43.2933) -> (152.9077, -43.566)
  line L2587 (153.3158, -45.6181) -> (153.7973, -45.7138)
  line L2588 (153.7973, -45.7138) -> (154.2788, -45.6181)
  line L2589 (152.5392, -44.4557) -> (152.6349, -44.9372)
  line L2590 (152.6349, -44.9372) -> (152.9077, -45.3453)
  line L2591 (153.7973, -43.1975) -> (153.3158, -43.2933)
  line L2592 (152.9077, -43.566) -> (152.6349, -43.9742)
  line L2593 (152.6349, -43.9742) -> (152.5392, -44.4557)
  line L2594 (152.9077, -45.3453) -> (153.3158, -45.6181)
  line L2595 (154.6869, -45.3453) -> (154.9597, -44.9372)
  line L2596 (154.2788, -45.6181) -> (154.6869, -45.3453)
  line L2597 (154.9597, -43.9742) -> (154.6869, -43.566)
  line L2598 (154.2788, -43.2933) -> (153.7973, -43.1975)
  line L2599 (154.6869, -43.566) -> (154.2788, -43.2933)
  line L2600 (154.9597, -44.9372) -> (155.0554, -44.4557)
  line L2601 (155.0554, -44.4557) -> (154.9597, -43.9742)
  line L2602 (171.4183, -16.9304) -> (170.8263, -17.3846)
  line L2603 (175.3226, -20.8347) -> (175.6081, -20.1454)
  line L2604 (173.5871, -22.1664) -> (174.2764, -21.8809)
  line L2605 (174.2764, -21.8809) -> (174.8684, -21.4267)
  line L2606 (170.8263, -21.4267) -> (171.4183, -21.8809)
  line L2607 (174.8684, -17.3846) -> (174.2764, -16.9304)
  line L2608 (170.0866, -18.6659) -> (169.9892, -19.4056)
  line L2609 (170.0866, -20.1454) -> (170.3721, -20.8347)
  line L2610 (172.1076, -16.6449) -> (171.4183, -16.9304)
  line L2611 (171.4183, -21.8809) -> (172.1076, -22.1664)
  line L2612 (170.3721, -17.9766) -> (170.0866, -18.6659)
  line L2613 (172.8473, -22.2638) -> (173.5871, -22.1664)
  line L2614 (175.6081, -18.6659) -> (175.3226, -17.9766)
  line L2615 (170.8263, -17.3846) -> (170.3721, -17.9766)
  line L2616 (172.1076, -22.1664) -> (172.8473, -22.2638)
  line L2617 (175.6081, -20.1454) -> (175.7055, -19.4056)
  line L2618 (174.2764, -16.9304) -> (173.5871, -16.6449)
  line L2619 (175.7055, -19.4056) -> (175.6081, -18.6659)
  line L2620 (169.9892, -19.4056) -> (170.0866, -20.1454)
  line L2621 (172.8473, -16.5475) -> (172.1076, -16.6449)
  line L2622 (173.5871, -16.6449) -> (172.8473, -16.5475)
  line L2623 (175.3226, -17.9766) -> (174.8684, -17.3846)
  line L2624 (170.3721, -20.8347) -> (170.8263, -21.4267)
  line L2625 (174.8684, -21.4267) -> (175.3226, -20.8347)
  line L2626 (170.3721, -78.0102) -> (170.8263, -78.6022)
  line L2627 (172.1076, -79.3419) -> (172.8473, -79.4393)
  line L2628 (175.3226, -75.1521) -> (174.8684, -74.5601)
  line L2629 (171.4183, -74.1059) -> (170.8263, -74.5601)
  line L2630 (174.2764, -74.1059) -> (173.5871, -73.8204)
  line L2631 (170.3721, -75.1521) -> (170.0866, -75.8414)
  line L2632 (169.9892, -76.5812) -> (170.0866, -77.3209)
  line L2633 (175.3226, -78.0102) -> (175.6081, -77.3209)
  line L2634 (170.0866, -77.3209) -> (170.3721, -78.0102)
  line L2635 (172.8473, -79.4393) -> (173.5871, -79.3419)
  line L2636 (171.4183, -79.0564) -> (172.1076, -79.3419)
  line L2637 (170.8263, -78.6022) -> (171.4183, -79.0564)
  line L2638 (175.6081, -77.3209) -> (175.7055, -76.5812)
  line L2639 (175.6081, -75.8414) -> (175.3226, -75.1521)
  line L2640 (173.5871, -79.3419) -> (174.2764, -79.0564)
  line L2641 (174.8684, -74.5601) -> (174.2764, -74.1059)
  line L2642 (170.0866, -75.8414) -> (169.9892, -76.5812)
  line L2643 (174.8684, -78.6022) -> (175.3226, -78.0102)
  line L2644 (170.8263, -74.5601) -> (170.3721, -75.1521)
  line L2645 (172.1076, -73.8204) -> (171.4183, -74.1059)
  line L2646 (173.5871, -73.8204) -> (172.8473, -73.723)
  line L2647 (174.2764, -79.0564) -> (174.8684, -78.6022)
  line L2648 (172.8473, -73.723) -> (172.1076, -73.8204)
  line L2649 (175.7055, -76.5812) -> (175.6081, -75.8414)
  line L2650 (175.6081, -37.7159) -> (175.3226, -37.0266)
  line L2651 (174.8684, -40.4767) -> (175.3226, -39.8847)
  line L2652 (172.1076, -41.2164) -> (172.8473, -41.3138)
  line L2653 (175.6081, -39.1954) -> (175.7055, -38.4557)
  line L2654 (174.2764, -35.9805) -> (173.5871, -35.6949)
  line L2655 (170.0866, -37.7159) -> (169.9892, -38.4557)
  line L2656 (170.3721, -37.0266) -> (170.0866, -37.7159)
  line L2657 (174.8684, -36.4347) -> (174.2764, -35.9805)
  line L2658 (169.9892, -38.4557) -> (170.0866, -39.1954)
  line L2659 (175.3226, -39.8847) -> (175.6081, -39.1954)
  line L2660 (170.0866, -39.1954) -> (170.3721, -39.8847)
  line L2661 (170.3721, -39.8847) -> (170.8263, -40.4767)
  line L2662 (172.1076, -35.6949) -> (171.4183, -35.9805)
  line L2663 (171.4183, -40.9309) -> (172.1076, -41.2164)
  line L2664 (174.2764, -40.9309) -> (174.8684, -40.4767)
  line L2665 (173.5871, -35.6949) -> (172.8473, -35.5975)
  line L2666 (170.8263, -36.4347) -> (170.3721, -37.0266)
  line L2667 (175.3226, -37.0266) -> (174.8684, -36.4347)
  line L2668 (172.8473, -35.5975) -> (172.1076, -35.6949)
  line L2669 (172.8473, -41.3138) -> (173.5871, -41.2164)
  line L2670 (173.5871, -41.2164) -> (174.2764, -40.9309)
  line L2671 (175.7055, -38.4557) -> (175.6081, -37.7159)
  line L2672 (171.4183, -35.9805) -> (170.8263, -36.4347)
  line L2673 (170.8263, -40.4767) -> (171.4183, -40.9309)
  line L2674 (170.8263, -59.5394) -> (171.4183, -59.9936)
  line L2675 (175.3226, -56.0893) -> (174.8684, -55.4974)
  line L2676 (173.5871, -60.2792) -> (174.2764, -59.9936)
  line L2677 (170.8263, -55.4974) -> (170.3721, -56.0893)
  line L2678 (175.6081, -58.2582) -> (175.7055, -57.5184)
  line L2679 (172.8473, -60.3766) -> (173.5871, -60.2792)
  line L2680 (174.2764, -59.9936) -> (174.8684, -59.5394)
  line L2681 (172.1076, -60.2792) -> (172.8473, -60.3766)
  line L2682 (170.0866, -56.7787) -> (169.9892, -57.5184)
  line L2683 (170.3721, -56.0893) -> (170.0866, -56.7787)
  line L2684 (171.4183, -59.9936) -> (172.1076, -60.2792)
  line L2685 (169.9892, -57.5184) -> (170.0866, -58.2582)